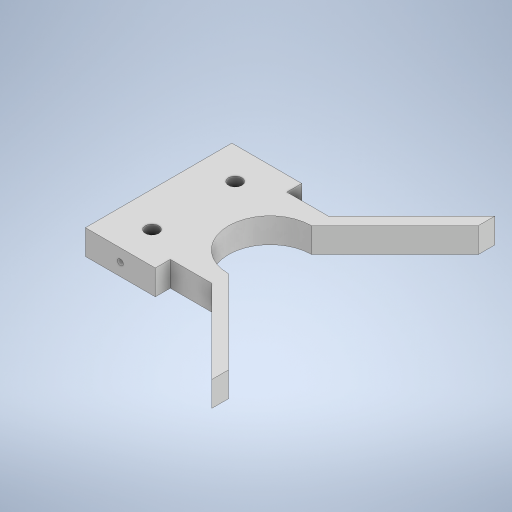
# Autodesk Inventor part: bas
Saved by Autodesk Inventor 2024.1 (Build 281209000, 209)
## iProperties
Created: 2024-04-06
Part Number: bas
Material: Générique
Document SubType Name: Modeling
Designer: chass
Density: 1 g/cm^3
Appearance: Par défaut
Author: chass
Autodesk Inventor part; units mm, degrees
ref_plane "YZ Plane" through (0, 0, 0) normal (1, 0, 0) x (0, 1, 0)
ref_plane "XZ Plane" through (0, 0, 0) normal (0, 1, 0) x (-1, 0, 0)
ref_plane "XY Plane" through (0, 0, 0) normal (0, 0, 1) x (1, 0, 0)
sketch "Esquisse1" plane through (0, 0, 0) normal (0, 1, 0) x (-1, 0, 0)
  line L0 (21, 44) -> (-21, 44)
  line L1 (-21, 44) -> (-21, -44)
  line L2 (-21, -44) -> (21, -44)
  line L3 (21, -44) -> (21, 44)
  line L4 (21, 44) -> (-21, -44)
  line L5 (-21, 44) -> (21, -44)
  circle A0 centre (0, 25) radius 4.05
  line L6 (21, 0) -> (-21, 0)
  circle A1 centre (0, -25) radius 4.05
  point P0 (0, 0)
  point P1 (0, 0)
  point P2 (0, 0)
  dimension "d0" = 88
  dimension "d1" = 42
  dimension "d2" = 8.1
  dimension "d3" = 25
  constraints: 14 end point, 4 midpoint, 2 centre point, 2 parallel, 1 coincident, 1 horizontal, 1 perpendicular, 1 symmetric about line, 1 other
  measures "d0" distance of L2.end L0.start
  measures "d1" distance of L1.end L2.end
  measures "d2" diameter of A0
  measures "d3" distance of point (0, 0) A0.centre
extrude "Extrusion1" add sketch "Esquisse1" along normal blind 15
sketch "Esquisse2" plane through (-21, 0, 44) normal (0, 0, 1) x (1, 0, 0)
  circle A0 centre (21, 7.5) radius 1.75
  line L0 (0, 0) -> (42, 0) projected
  point P0 (21, 0)
  point P1 (21, 0)
  dimension "d6" = 7.5
  dimension "d7" = 3.5
  constraints: 1 centre point, 1 midpoint
  measures "d6" distance of point (21, 0) A0.centre
  measures "d7" diameter of A0
extrude "Extrusion2" cut sketch "Esquisse2" against normal blind 16
sketch "Esquisse3" plane through (21, 0, -44) normal (0, 0, -1) x (-1, 0, 0)
  circle A0 centre (21, 7.5) radius 1.75 projected
  circle A1 centre (21, 7.5) radius 1.75
  point P0 (21, 0)
  constraints: 1 centre point, 1 coincident
extrude "Extrusion3" cut sketch "Esquisse3" against normal blind 16
sketch "Esquisse4" plane through (0, 0, 0) normal (0, -1, 0) x (1, 0, 0)
  circle A0 centre (46, 0) radius 25
  line L0 (21, 44) -> (21, -44) projected
  line L1 (46, 25) -> (21, 25)
  line L2 (21, 35) -> (46, 35)
  line L3 (46, 35) -> (96, 85)
  line L4 (46, 35) -> (116.7107, 35) construction
  line L5 (96, 85) -> (96, 75)
  line L6 (96, 75) -> (46, 25)
  line L7 (21, 0) -> (110, 0)
  line L8 (46, -25) -> (21, -25)
  line L9 (21, -35) -> (46, -35)
  line L10 (46, -35) -> (96, -85)
  line L11 (96, -85) -> (96, -75)
  line L12 (96, -75) -> (46, -25)
  point P0 (0, 0)
  point P1 (46, -25)
  point P2 (21, 0)
  dimension "d12" = 50
  dimension "d13" = 25
  dimension "d14" = 10
  dimension "d15" = 45
  dimension "d16" = 50
  dimension "d17" = 10
  constraints: 24 end point, 7 symmetric about line, 3 horizontal, 2 point on circle, 2 point on line, 1 centre point, 1 equal length, 1 midpoint, 1 perpendicular, 1 vertical
  measures "d12" diameter of A0
  measures "d13" distance from line of L0 A0.centre
  measures "d14" distance between parallel lines of L1 L2
  measures "d15" angle of L4 L3
  measures "d16" horizontal distance of L2.end L3.end
  measures "d17" distance of L3.end L5.end
extrude "Extrusion4" add sketch "Esquisse4" against normal blind 15 contours A0 L0 L1 | L1 L0 L2 L3 L5 L6 | L8 L0 A0 | L12 L11 L10 L9 L0 L8
